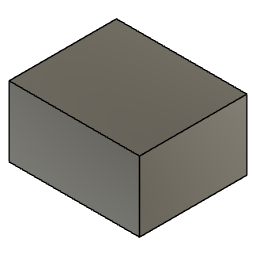
배터리 (Autodesk Fusion 360 design; units mm, degrees)
Autodesk Fusion 360 part; units mm, degrees
sketch "스케치1" plane through (0, 0, 0) normal (0, 0, 1) x (1, 0, 0)
  line L0 (-40.8158, 37.5935) -> (89.1842, 37.5935)
  line L1 (89.1842, 37.5935) -> (89.1842, -69.4065)
  line L2 (89.1842, -69.4065) -> (-40.8158, -69.4065)
  line L3 (-40.8158, -69.4065) -> (-40.8158, 37.5935)
  dimension "d1" = 130
  dimension "d2" = 107
  constraint horizontal L0
  constraint vertical L1
  constraint horizontal L2
  constraint vertical L3
  measures "d1" distance of L0.start L0.end
  measures "d2" distance of L0.start L2.end
extrude "돌출1" add sketch "스케치1" along normal blind 70
